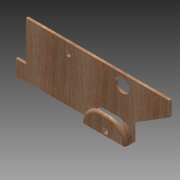
# Autodesk Inventor part: Shooter_TopMotorSupport
Saved by Autodesk Inventor 2014 (Build 180170000, 170)
## iProperties
Created: 2016-01-26
Part Number: Shooter_TopMotorSupport
Material: Generic
Document SubType Name: Modeling
Designer: choices
Density: 1 g/cm^3
Appearance: Birch - Natural Polished
Author: choices
Autodesk Inventor part; units mm, degrees
ref_plane "YZ Plane" through (0, 0, 0) normal (1, 0, 0) x (0, 1, 0)
ref_plane "XZ Plane" through (0, 0, 0) normal (0, 1, 0) x (-1, 0, 0)
ref_plane "XY Plane" through (0, 0, 0) normal (0, 0, 1) x (1, 0, 0)
sketch "Sketch1" plane through (0, 0, 0) normal (0, 0, 1) x (1, 0, 0)
  circle A0 centre (0, 0) radius 12.7
  circle A1 centre (0, 0) radius 50.8
  line L0 (50.8, 0) -> (50.8, -225.3234)
  line L1 (50.8, -225.3234) -> (-50.8, -225.3234)
  line L2 (-50.8, -225.3234) -> (-50.8, 0)
  line L3 (-50.8, 0) -> (-12.7, 0)
  line L4 (12.7, 0) -> (50.8, 0)
  dimension "d1" = 101.6
  dimension "d0" = 25.4
  dimension "d2" = 225.3234
  constraints: 10 end point, 3 parallel, 2 coincident, 2 horizontal, 2 perpendicular, 2 point on circle, 1 centre point, 1 horizontal alignment, 2 other
  measures "d0" diameter of A0
  measures "d2" distance of L0.start L0.end
extrude "Extrusion1" add sketch "Sketch1" along normal blind 12.7 contours L4 A1 L3 A0 | A0 L3 A1 L4 | L0 L1 L2 A1
sketch "Sketch2" plane through (0, 0, 12.7) normal (0, 0, 1) x (1, 0, 0)
  circle A0 centre (0, 0) radius 12.7 projected
  arc A1 (50.8, 0) -> (-50.8, 0) centre (0, 0) ccw projected
  line L0 (-50.8, 0) -> (-50.8, -225.3234) projected
  line L1 (-50.8, -225.3234) -> (50.8, -225.3234) projected
  line L2 (50.8, -225.3234) -> (50.8, 0) projected
  circle A2 centre (176.5046, -179.1208) radius 32.385
  circle A3 centre (253.9746, -179.1208) radius 32.385
  line L3 (144.1196, -225.3234) -> (144.1196, -179.1208)
  line L4 (286.3596, -225.3234) -> (286.3596, -179.1208)
  line L5 (176.5046, -146.7358) -> (253.9746, -146.7358)
  line L6 (50.8, -225.3234) -> (144.1196, -225.3234)
  line L7 (286.3596, -225.3234) -> (508, -225.3234)
  line L8 (-50.8, -225.3234) -> (-238.2266, -225.3234)
  line L9 (-263.6266, -225.3234) -> (-263.6266, -150.876)
  line L10 (-263.6266, -150.876) -> (-212.8266, -150.876)
  line L11 (-212.8266, -150.876) -> (-212.8266, 50.8)
  line L12 (-212.8266, 50.8) -> (508, 50.8)
  line L13 (508, 50.8) -> (508, -225.3234)
  line L14 (-238.2266, -229.108) -> (-238.2266, -225.3234)
  line L15 (-238.2266, -229.108) -> (-263.6266, -229.108)
  line L16 (-263.6266, -229.108) -> (-263.6266, -225.3234)
  dimension "d5" = 176.5046
  dimension "d6" = 179.1208
  dimension "d7" = 64.77
  dimension "d8" = 64.77
  dimension "d9" = 77.47
  dimension "d11" = 212.8266
  dimension "d13" = 50.8
  dimension "d16" = 150.876
  dimension "d17" = 508
  dimension "d18" = 229.108
  constraints: 28 end point, 8 perpendicular, 4 point on circle, 3 parallel, 2 centre point, 2 tangent, 1 coincident, 1 collinear
  measures "d5" horizontal distance of point (176.505, -179.121) A0.centre
  measures "d6" vertical distance of A0.centre point (176.505, -179.121)
  measures "d7" diameter of A2
  measures "d8" diameter of A3
  measures "d9" distance of point (176.505, -179.121) A3.centre
  measures "d11" distance of L0.end L9.start
  measures "d13" distance of L9.end L10.end
  measures "d16" distance from line of A0.centre L10
  measures "d17" distance from line of L13 A0.centre
  measures "d18" vertical distance of L14.start A1.centre
extrude "Extrusion2" add sketch "Sketch2" against normal blind 12.7 contours A1 L12 L13 L7 L4 A3 L5 A2 L3 L6 L2 | A1 L0 L8 L14 L15 L16 L9 L10 L11 L12
sketch "Sketch3" plane through (0, 0, 12.7) normal (0, 0, 1) x (1, 0, 0)
  circle A0 centre (0, 0) radius 12.7 projected
  circle A1 centre (225.0958, -205.5114) radius 12.7
  dimension "d19" = 25.4
  dimension "d20" = 304.8
  dimension "d21" = 205.5114
  constraints: 1 centre point
  measures "d19" diameter of A1
  measures "d20" distance of A1.centre A0.centre
  measures "d21" vertical distance of A1.centre A0.centre
sketch "Sketch4" plane through (0, 0, 12.7) normal (0, 0, 1) x (1, 0, 0)
  line L0 (144.1196, -225.3234) -> (106.0196, -225.3234)
  line L1 (106.0196, -225.3234) -> (106.0196, -136.4234)
  line L2 (106.0196, -136.4234) -> (144.1196, -136.4234)
  line L3 (144.1196, -136.4234) -> (144.1196, -225.3234)
  line L4 (286.3596, -225.3234) -> (324.4596, -225.3234)
  line L5 (324.4596, -225.3234) -> (324.4596, -136.4234)
  line L6 (324.4596, -136.4234) -> (286.3596, -136.4234)
  line L7 (286.3596, -136.4234) -> (286.3596, -225.3234)
  dimension "d22" = 38.1
  dimension "d23" = 88.9
  dimension "d24" = 38.1
  dimension "d25" = 88.9
  constraints: 16 end point, 4 parallel, 2 horizontal, 2 perpendicular
  measures "d22" distance of L1.end L2.end
  measures "d23" distance of L0.end L1.end
  measures "d24" distance of L6.end L5.end
  measures "d25" distance of L5.end L4.end
extrude "Extrusion3" add sketch "Sketch4" along normal blind 25.4
sketch "Sketch5" plane through (0, 0, 38.1) normal (0, 0, 1) x (1, 0, 0)
  line L0 (106.0196, -136.4234) -> (324.4596, -136.4234)
  line L1 (324.4596, -136.4234) -> (324.4596, -225.3234)
  line L2 (324.4596, -225.3234) -> (106.0196, -225.3234)
  line L3 (106.0196, -225.3234) -> (106.0196, -136.4234)
  point P0 (0, 0)
  dimension "d28" = 218.44
  constraints: 8 end point, 2 parallel, 1 horizontal, 1 perpendicular
  measures "d28" distance of L1.end L2.end
extrude "Extrusion4" add sketch "Sketch5" along normal blind 12.7
extrude "Extrusion5" cut sketch "Sketch3" along normal blind 76.2 contours A1
sketch "Sketch6" plane through (0, 0, 12.7) normal (0, 0, 1) x (1, 0, 0)
  line L0 (324.4596, -136.4234) -> (324.4596, -225.3234) projected
  line L1 (324.4596, -225.3234) -> (508, -225.3234) projected
  line L2 (508, -225.3234) -> (508, 50.8) projected
  line L3 (324.4596, -136.4234) -> (508, -22.1234)
  dimension "d33" = 203.2
  constraints: 2 end point, 1 point on line
  measures "d33" distance from line of L1 L3.end
extrude "Extrusion6" cut sketch "Sketch6" against normal blind 25.4
sketch "Sketch7" plane through (0, 0, 50.8) normal (0, 0, 1) x (1, 0, 0)
  line L0 (106.0196, -136.4234) -> (106.0196, -225.3234) projected
  line L1 (324.4596, -225.3234) -> (324.4596, -136.4234) projected
  line L2 (324.4596, -136.4234) -> (106.0196, -136.4234) projected
  arc A0 (324.4596, -225.3234) -> (235.5596, -136.4234) centre (235.5596, -225.3234) ccw
  line L3 (324.4596, -225.3234) -> (235.5596, -136.4234) construction
  line L4 (324.4596, -225.3234) -> (450.1832, -225.3234) construction
  arc A1 (194.9196, -136.4234) -> (106.0196, -225.3234) centre (194.9196, -225.3234) ccw
  line L5 (106.0196, -225.3234) -> (194.9196, -136.4234) construction
  line L6 (106.0196, -225.3234) -> (231.7432, -225.3234) construction
  point P0 (0, 0)
  dimension "d36" = 135
  dimension "d37" = 45
  constraints: 8 end point, 4 point on circle, 4 tangent, 2 centre point, 2 equal length, 2 horizontal, 2 point on line
  measures "d36" angle of L4 L3
  measures "d37" angle of L6 L5
extrude "Extrusion7" cut sketch "Sketch7" against normal blind 38.1
fillet "Fillet1" radius 12.7 3 edges at (215.2396, -136.4234, 50.8) (298.4214, -162.4616, 50.8) (132.0578, -162.4616, 50.8)
sketch "Sketch8" plane through (0, 0, 0) normal (0, 0, -1) x (-1, 0, 0)
  line L0 (-508, 50.8) -> (-508, -22.1234) projected
  circle A0 centre (0, 0) radius 12.7 projected
  line L1 (0, 0) -> (-271.2669, 0)
  circle A1 centre (-271.2669, 0) radius 35.56
  dimension "d41" = 71.12
  constraints: 2 end point, 1 centre point, 1 coincident, 1 perpendicular
  measures "d41" diameter of A1
extrude "Extrusion8" cut sketch "Sketch8" against normal blind 25.4 contours A1
sketch "Sketch9" plane through (0, 0, 0) normal (0, 0, -1) x (-1, 0, 0)
  circle A0 centre (-271.2669, 0) radius 35.56 projected
  line L0 (-324.4596, -136.4234) -> (-324.4596, -225.3234) projected
  line L1 (-324.4596, -225.3234) -> (-286.3596, -225.3234) projected
  line L2 (-286.3596, -225.3234) -> (-286.3596, -179.1208) projected
  arc A1 (-253.9746, -146.7358) -> (-286.3596, -179.1208) centre (-253.9746, -179.1208) ccw projected
  line L3 (-253.9746, -146.7358) -> (-176.5046, -146.7358) projected
  arc A2 (-144.1196, -179.1208) -> (-176.5046, -146.7358) centre (-176.5046, -179.1208) ccw projected
  line L4 (-144.1196, -179.1208) -> (-144.1196, -225.3234) projected
  line L5 (-144.1196, -225.3234) -> (238.2266, -225.3234) projected
  line L6 (238.2266, -225.3234) -> (238.2266, -229.108) projected
  line L7 (238.2266, -229.108) -> (263.6266, -229.108) projected
  line L8 (263.6266, -229.108) -> (263.6266, -150.876) projected
  line L9 (263.6266, -150.876) -> (212.8266, -150.876) projected
  line L10 (212.8266, -150.876) -> (212.8266, 50.8) projected
  line L11 (212.8266, 50.8) -> (-508, 50.8) projected
  line L12 (-508, 50.8) -> (-508, -22.1234) projected
  line L13 (-508, -22.1234) -> (-324.4596, -136.4234) projected
  circle A3 centre (0, 0) radius 12.7 projected
body "Solid1"
